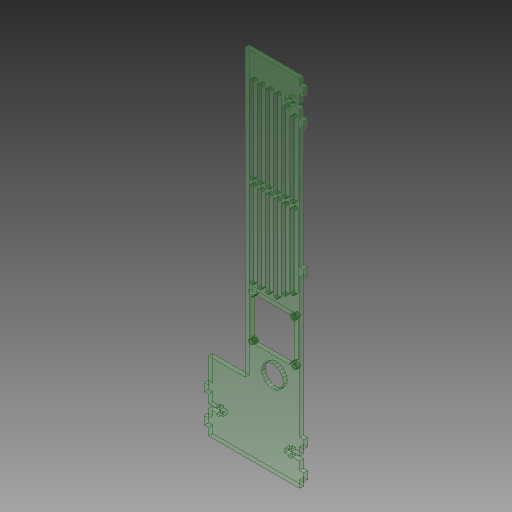
# Autodesk Inventor part: EE Side 2
Saved by Autodesk Inventor 2018 (Build 220112000, 112)
## iProperties
Created: 2016-07-27
Part Number: EE Side 2
Material: Polycarbonate, Green
Document SubType Name: Modeling
Designer: User
Density: 1.2 g/cm^3
Appearance: Polycarbonate - Clear(2)
Author: User
Autodesk Inventor part; units mm, degrees
ref_plane "YZ Plane" through (0, 0, 0) normal (1, 0, 0) x (0, 1, 0)
ref_plane "XZ Plane" through (0, 0, 0) normal (0, 1, 0) x (-1, 0, 0)
ref_plane "XY Plane" through (0, 0, 0) normal (0, 0, 1) x (1, 0, 0)
sketch "Sketch1" plane through (0, 0, 0) normal (0, 0, 1) x (1, 0, 0)
  line L0 (150.9594, -29.9434) -> (150.9594, -23.8434)
  line L1 (150.9594, -23.8434) -> (153.9594, -23.8434)
  line L2 (153.9594, -23.8434) -> (153.9594, -17.8434)
  line L3 (153.9594, -17.8434) -> (150.9594, -17.8434)
  line L4 (150.9594, -17.8434) -> (150.9594, -13.3231)
  line L5 (150.9594, -13.3231) -> (146.9594, -13.3231)
  line L6 (146.9594, -13.3231) -> (143.9594, -13.3231)
  line L7 (143.9594, -13.3231) -> (140.9594, -13.3231)
  line L8 (140.9594, -13.3231) -> (137.9594, -13.3231)
  line L9 (137.9594, -13.3231) -> (134.9594, -13.3231)
  line L10 (134.9594, -13.3231) -> (131.9593, -13.3231)
  line L11 (131.9593, -13.3231) -> (128.9594, -13.3231)
  line L12 (128.9594, -13.3231) -> (125.9593, -13.3231)
  line L13 (125.9593, -13.3231) -> (122.9594, -13.3231)
  line L14 (122.9594, -13.3231) -> (119.9594, -13.3231)
  line L15 (119.9594, -13.3231) -> (116.9593, -13.3231)
  line L16 (116.9593, -13.3231) -> (113.9593, -13.3231)
  line L17 (113.9593, -13.3231) -> (110.9594, -13.3231)
  line L18 (110.9594, -13.3231) -> (110.9594, -118.3231)
  line L19 (110.9594, -118.3231) -> (110.9594, -223.7405)
  line L20 (110.9594, -223.7405) -> (83.9593, -223.7405)
  line L21 (83.9593, -223.7405) -> (83.9593, -242.1298)
  line L22 (83.9593, -242.1298) -> (80.9594, -242.1298)
  line L23 (80.9594, -242.1298) -> (80.9594, -248.1298)
  line L24 (80.9594, -248.1298) -> (83.9593, -248.1298)
  line L25 (83.9593, -248.1298) -> (83.9593, -250.7405)
  line L26 (83.9593, -250.7405) -> (83.9593, -254.2298)
  line L27 (83.9593, -254.2298) -> (89.9593, -254.2298)
  line L28 (89.9593, -254.2298) -> (89.9593, -252.9798)
  line L29 (89.9593, -252.9798) -> (91.9594, -252.9798)
  line L30 (91.9594, -252.9798) -> (91.9594, -254.2298)
  line L31 (91.9594, -254.2298) -> (94.6093, -254.2298)
  line L32 (94.6093, -254.2298) -> (94.6093, -257.2298)
  line L33 (94.6093, -257.2298) -> (91.9594, -257.2298)
  line L34 (91.9594, -257.2298) -> (91.9594, -258.4798)
  line L35 (91.9594, -258.4798) -> (89.9593, -258.4798)
  line L36 (89.9593, -258.4798) -> (89.9593, -257.2298)
  line L37 (89.9593, -257.2298) -> (83.9593, -257.2298)
  line L38 (83.9593, -257.2298) -> (83.9593, -263.3298)
  line L39 (83.9593, -263.3298) -> (80.9594, -263.3298)
  line L40 (80.9594, -263.3298) -> (80.9594, -269.3297)
  line L41 (80.9594, -269.3297) -> (83.9593, -269.3297)
  line L42 (83.9593, -269.3297) -> (83.9593, -269.4298)
  line L43 (83.9593, -269.4298) -> (83.9593, -274.7405)
  line L44 (83.9593, -274.7405) -> (150.9594, -274.7405)
  line L45 (150.9594, -274.7405) -> (150.9594, -269.3434)
  line L46 (150.9594, -269.3434) -> (153.9594, -269.3434)
  line L47 (153.9594, -269.3434) -> (153.9594, -263.3434)
  line L48 (153.9594, -263.3434) -> (150.9594, -263.3434)
  line L49 (150.9594, -263.3434) -> (150.9594, -260.7327)
  line L50 (150.9594, -260.7327) -> (150.9594, -257.2434)
  line L51 (150.9594, -257.2434) -> (144.9593, -257.2434)
  line L52 (144.9593, -257.2434) -> (144.9593, -258.4934)
  line L53 (144.9593, -258.4934) -> (142.9593, -258.4934)
  line L54 (142.9593, -258.4934) -> (142.9593, -257.2434)
  line L55 (142.9593, -257.2434) -> (140.3094, -257.2434)
  line L56 (140.3094, -257.2434) -> (140.3094, -254.2434)
  line L57 (140.3094, -254.2434) -> (142.9593, -254.2434)
  line L58 (142.9593, -254.2434) -> (142.9593, -252.9934)
  line L59 (142.9593, -252.9934) -> (144.9593, -252.9934)
  line L60 (144.9593, -252.9934) -> (144.9593, -254.2434)
  line L61 (144.9593, -254.2434) -> (150.9594, -254.2434)
  line L62 (150.9594, -254.2434) -> (150.9594, -248.1434)
  line L63 (150.9594, -248.1434) -> (153.9594, -248.1434)
  line L64 (153.9594, -248.1434) -> (153.9594, -242.1434)
  line L65 (153.9594, -242.1434) -> (150.9594, -242.1434)
  line L66 (150.9594, -242.1434) -> (150.9594, -139.5434)
  line L67 (150.9594, -139.5434) -> (153.9594, -139.5434)
  line L68 (153.9594, -139.5434) -> (153.9594, -133.5434)
  line L69 (153.9594, -133.5434) -> (150.9594, -133.5434)
  line L70 (150.9594, -133.5434) -> (150.9594, -45.0434)
  line L71 (150.9594, -45.0434) -> (153.9594, -45.0434)
  line L72 (153.9594, -45.0434) -> (153.9594, -39.0434)
  line L73 (153.9594, -39.0434) -> (150.9594, -39.0434)
  line L74 (150.9594, -39.0434) -> (150.9594, -36.4327)
  line L75 (150.9594, -36.4327) -> (150.9594, -32.9434)
  line L76 (150.9594, -32.9434) -> (144.9593, -32.9434)
  line L77 (144.9593, -32.9434) -> (144.9593, -34.1934)
  line L78 (144.9593, -34.1934) -> (142.9593, -34.1934)
  line L79 (142.9593, -34.1934) -> (142.9593, -32.9434)
  line L80 (142.9593, -32.9434) -> (140.3094, -32.9434)
  line L81 (140.3094, -32.9434) -> (140.3094, -29.9434)
  line L82 (140.3094, -29.9434) -> (142.9593, -29.9434)
  line L83 (142.9593, -29.9434) -> (142.9593, -28.6934)
  line L84 (142.9593, -28.6934) -> (144.9593, -28.6934)
  line L85 (144.9593, -28.6934) -> (144.9593, -29.9434)
  line L86 (144.9593, -29.9434) -> (150.9594, -29.9434)
  line L87 (146.5595, -170.5352) -> (146.17, -170.4202)
  line L88 (146.17, -170.4202) -> (145.7956, -170.2628)
  line L89 (145.7956, -170.2628) -> (145.4409, -170.065)
  line L90 (145.4409, -170.065) -> (145.1102, -169.8292)
  line L91 (145.1102, -169.8292) -> (144.8075, -169.5584)
  line L92 (144.8075, -169.5584) -> (144.5367, -169.2558)
  line L93 (144.5367, -169.2558) -> (144.3009, -168.925)
  line L94 (144.3009, -168.925) -> (144.1031, -168.5703)
  line L95 (144.1031, -168.5703) -> (143.9458, -168.1959)
  line L96 (143.9458, -168.1959) -> (143.8307, -167.8064)
  line L97 (143.8307, -167.8064) -> (143.7593, -167.4066)
  line L98 (143.7593, -167.4066) -> (118.1593, -167.4066)
  line L99 (118.1593, -167.4066) -> (118.0788, -167.8022)
  line L100 (118.0788, -167.8022) -> (117.9568, -168.1871)
  line L101 (117.9568, -168.1871) -> (117.7946, -168.5569)
  line L102 (117.7946, -168.5569) -> (117.5941, -168.9073)
  line L103 (117.5941, -168.9073) -> (117.3575, -169.2346)
  line L104 (117.3575, -169.2346) -> (117.0876, -169.5348)
  line L105 (117.0876, -169.5348) -> (116.7874, -169.8048)
  line L106 (116.7874, -169.8048) -> (116.4601, -170.0413)
  line L107 (116.4601, -170.0413) -> (116.1097, -170.2418)
  line L108 (116.1097, -170.2418) -> (115.7399, -170.404)
  line L109 (115.7399, -170.404) -> (115.355, -170.5261)
  line L110 (115.355, -170.5261) -> (114.9593, -170.6066)
  line L111 (114.9593, -170.6066) -> (114.9593, -196.2066)
  line L112 (114.9593, -196.2066) -> (115.3592, -196.2779)
  line L113 (115.3592, -196.2779) -> (115.7487, -196.393)
  line L114 (115.7487, -196.393) -> (116.1231, -196.5503)
  line L115 (116.1231, -196.5503) -> (116.4778, -196.7482)
  line L116 (116.4778, -196.7482) -> (116.8085, -196.9839)
  line L117 (116.8085, -196.9839) -> (117.1111, -197.2548)
  line L118 (117.1111, -197.2548) -> (117.382, -197.5574)
  line L119 (117.382, -197.5574) -> (117.6178, -197.8881)
  line L120 (117.6178, -197.8881) -> (117.8156, -198.2428)
  line L121 (117.8156, -198.2428) -> (117.9729, -198.6172)
  line L122 (117.9729, -198.6172) -> (118.088, -199.0067)
  line L123 (118.088, -199.0067) -> (118.1593, -199.4066)
  line L124 (118.1593, -199.4066) -> (143.7593, -199.4066)
  line L125 (143.7593, -199.4066) -> (143.8399, -199.0109)
  line L126 (143.8399, -199.0109) -> (143.9619, -198.626)
  line L127 (143.9619, -198.626) -> (144.1241, -198.2563)
  line L128 (144.1241, -198.2563) -> (144.3246, -197.9058)
  line L129 (144.3246, -197.9058) -> (144.5611, -197.5786)
  line L130 (144.5611, -197.5786) -> (144.8311, -197.2783)
  line L131 (144.8311, -197.2783) -> (145.1314, -197.0084)
  line L132 (145.1314, -197.0084) -> (145.4586, -196.7718)
  line L133 (145.4586, -196.7718) -> (145.8091, -196.5713)
  line L134 (145.8091, -196.5713) -> (146.1788, -196.4091)
  line L135 (146.1788, -196.4091) -> (146.5637, -196.2871)
  line L136 (146.5637, -196.2871) -> (146.9594, -196.2066)
  line L137 (146.9594, -196.2066) -> (146.9594, -170.6066)
  line L138 (146.9594, -170.6066) -> (146.5595, -170.5352)
  line L139 (148.6014, -198.9666) -> (148.4316, -198.5566)
  line L140 (148.4316, -198.5566) -> (148.1615, -198.2045)
  line L141 (148.1615, -198.2045) -> (147.8093, -197.9343)
  line L142 (147.8093, -197.9343) -> (147.3993, -197.7645)
  line L143 (147.3993, -197.7645) -> (146.9594, -197.7066)
  line L144 (146.9594, -197.7066) -> (146.5194, -197.7645)
  line L145 (146.5194, -197.7645) -> (146.1094, -197.9343)
  line L146 (146.1094, -197.9343) -> (145.7573, -198.2045)
  line L147 (145.7573, -198.2045) -> (145.4871, -198.5566)
  line L148 (145.4871, -198.5566) -> (145.3173, -198.9666)
  line L149 (145.3173, -198.9666) -> (145.2594, -199.4066)
  line L150 (145.2594, -199.4066) -> (145.3173, -199.8466)
  line L151 (145.3173, -199.8466) -> (145.4871, -200.2566)
  line L152 (145.4871, -200.2566) -> (145.7573, -200.6087)
  line L153 (145.7573, -200.6087) -> (146.1094, -200.8788)
  line L154 (146.1094, -200.8788) -> (146.5194, -201.0486)
  line L155 (146.5194, -201.0486) -> (146.9594, -201.1066)
  line L156 (146.9594, -201.1066) -> (147.3993, -201.0486)
  line L157 (147.3993, -201.0486) -> (147.8093, -200.8788)
  line L158 (147.8093, -200.8788) -> (148.1615, -200.6087)
  line L159 (148.1615, -200.6087) -> (148.4316, -200.2566)
  line L160 (148.4316, -200.2566) -> (148.6014, -199.8466)
  line L161 (148.6014, -199.8466) -> (148.6594, -199.4066)
  line L162 (148.6594, -199.4066) -> (148.6014, -198.9666)
  line L163 (148.6014, -166.9666) -> (148.4316, -166.5566)
  line L164 (148.4316, -166.5566) -> (148.1615, -166.2045)
  line L165 (148.1615, -166.2045) -> (147.8093, -165.9344)
  line L166 (147.8093, -165.9344) -> (147.3993, -165.7645)
  line L167 (147.3993, -165.7645) -> (146.9594, -165.7066)
  line L168 (146.9594, -165.7066) -> (146.5194, -165.7645)
  line L169 (146.5194, -165.7645) -> (146.1094, -165.9344)
  line L170 (146.1094, -165.9344) -> (145.7573, -166.2045)
  line L171 (145.7573, -166.2045) -> (145.4871, -166.5566)
  line L172 (145.4871, -166.5566) -> (145.3173, -166.9666)
  line L173 (145.3173, -166.9666) -> (145.2594, -167.4066)
  line L174 (145.2594, -167.4066) -> (145.3173, -167.8466)
  line L175 (145.3173, -167.8466) -> (145.4871, -168.2566)
  line L176 (145.4871, -168.2566) -> (145.7573, -168.6087)
  line L177 (145.7573, -168.6087) -> (146.1094, -168.8788)
  line L178 (146.1094, -168.8788) -> (146.5194, -169.0486)
  line L179 (146.5194, -169.0486) -> (146.9594, -169.1066)
  line L180 (146.9594, -169.1066) -> (147.3993, -169.0486)
  line L181 (147.3993, -169.0486) -> (147.8093, -168.8788)
  line L182 (147.8093, -168.8788) -> (148.1615, -168.6087)
  line L183 (148.1615, -168.6087) -> (148.4316, -168.2566)
  line L184 (148.4316, -168.2566) -> (148.6014, -167.8466)
  line L185 (148.6014, -167.8466) -> (148.6594, -167.4066)
  line L186 (148.6594, -167.4066) -> (148.6014, -166.9666)
  line L187 (116.6014, -198.9666) -> (116.4316, -198.5566)
  line L188 (116.4316, -198.5566) -> (116.1614, -198.2045)
  line L189 (116.1614, -198.2045) -> (115.8094, -197.9343)
  line L190 (115.8094, -197.9343) -> (115.3994, -197.7645)
  line L191 (115.3994, -197.7645) -> (114.9593, -197.7066)
  line L192 (114.9593, -197.7066) -> (114.5193, -197.7645)
  line L193 (114.5193, -197.7645) -> (114.1094, -197.9343)
  line L194 (114.1094, -197.9343) -> (113.7573, -198.2045)
  line L195 (113.7573, -198.2045) -> (113.4871, -198.5566)
  line L196 (113.4871, -198.5566) -> (113.3173, -198.9666)
  line L197 (113.3173, -198.9666) -> (113.2593, -199.4066)
  line L198 (113.2593, -199.4066) -> (113.3173, -199.8466)
  line L199 (113.3173, -199.8466) -> (113.4871, -200.2566)
  line L200 (113.4871, -200.2566) -> (113.7573, -200.6087)
  line L201 (113.7573, -200.6087) -> (114.1094, -200.8788)
  line L202 (114.1094, -200.8788) -> (114.5193, -201.0486)
  line L203 (114.5193, -201.0486) -> (114.9593, -201.1066)
  line L204 (114.9593, -201.1066) -> (115.3994, -201.0486)
  line L205 (115.3994, -201.0486) -> (115.8094, -200.8788)
  line L206 (115.8094, -200.8788) -> (116.1614, -200.6087)
  line L207 (116.1614, -200.6087) -> (116.4316, -200.2566)
  line L208 (116.4316, -200.2566) -> (116.6014, -199.8466)
  line L209 (116.6014, -199.8466) -> (116.6593, -199.4066)
  line L210 (116.6593, -199.4066) -> (116.6014, -198.9666)
  line L211 (116.9082, -32.9348) -> (116.7584, -32.5731)
  line L212 (116.7584, -32.5731) -> (116.52, -32.2624)
  line L213 (116.52, -32.2624) -> (116.2093, -32.024)
  line L214 (116.2093, -32.024) -> (115.8476, -31.8742)
  line L215 (115.8476, -31.8742) -> (115.4594, -31.8231)
  line L216 (115.4594, -31.8231) -> (115.0711, -31.8742)
  line L217 (115.0711, -31.8742) -> (114.7094, -32.024)
  line L218 (114.7094, -32.024) -> (114.3987, -32.2624)
  line L219 (114.3987, -32.2624) -> (114.1603, -32.5731)
  line L220 (114.1603, -32.5731) -> (114.0105, -32.9348)
  line L221 (114.0105, -32.9348) -> (113.9593, -33.3231)
  spline S0 degree 3 poles (113.9593, -33.3231) (113.9593, -53.8006) (113.8767, -74.2899) (114.0105, -94.7613) knots 11 11 11 11 12 12 12 12
  line L222 (113.9593, -33.3231) -> (113.9593, -53.8006) construction
  line L223 (113.9593, -53.8006) -> (113.8767, -74.2899) construction
  line L224 (113.8767, -74.2899) -> (114.0105, -94.7613) construction
  line L225 (114.0105, -94.7613) -> (114.1603, -95.1231)
  line L226 (114.1603, -95.1231) -> (114.3987, -95.4337)
  line L227 (114.3987, -95.4337) -> (114.7094, -95.6721)
  line L228 (114.7094, -95.6721) -> (115.0711, -95.822)
  line L229 (115.0711, -95.822) -> (115.4594, -95.8731)
  line L230 (115.4594, -95.8731) -> (115.8476, -95.822)
  line L231 (115.8476, -95.822) -> (116.2093, -95.6721)
  line L232 (116.2093, -95.6721) -> (116.52, -95.4337)
  line L233 (116.52, -95.4337) -> (116.7584, -95.1231)
  line L234 (116.7584, -95.1231) -> (116.9082, -94.7613)
  spline S1 degree 3 poles (116.9082, -94.7613) (117.0428, -74.1633) (117.0428, -53.5328) (116.9082, -32.9348) knots 22 22 22 22 23 23 23 23
  line L235 (116.9082, -94.7613) -> (117.0428, -74.1633) construction
  line L236 (117.0428, -74.1633) -> (117.0428, -53.5328) construction
  line L237 (117.0428, -53.5328) -> (116.9082, -32.9348) construction
  line L238 (116.6014, -166.9666) -> (116.4316, -166.5566)
  line L239 (116.4316, -166.5566) -> (116.1614, -166.2045)
  line L240 (116.1614, -166.2045) -> (115.8094, -165.9344)
  line L241 (115.8094, -165.9344) -> (115.3994, -165.7645)
  line L242 (115.3994, -165.7645) -> (114.9593, -165.7066)
  line L243 (114.9593, -165.7066) -> (114.5193, -165.7645)
  line L244 (114.5193, -165.7645) -> (114.1094, -165.9344)
  line L245 (114.1094, -165.9344) -> (113.7573, -166.2045)
  line L246 (113.7573, -166.2045) -> (113.4871, -166.5566)
  line L247 (113.4871, -166.5566) -> (113.3173, -166.9666)
  line L248 (113.3173, -166.9666) -> (113.2593, -167.4066)
  line L249 (113.2593, -167.4066) -> (113.3173, -167.8466)
  line L250 (113.3173, -167.8466) -> (113.4871, -168.2566)
  line L251 (113.4871, -168.2566) -> (113.7573, -168.6087)
  line L252 (113.7573, -168.6087) -> (114.1094, -168.8788)
  line L253 (114.1094, -168.8788) -> (114.5193, -169.0486)
  line L254 (114.5193, -169.0486) -> (114.9593, -169.1066)
  line L255 (114.9593, -169.1066) -> (115.3994, -169.0486)
  line L256 (115.3994, -169.0486) -> (115.8094, -168.8788)
  line L257 (115.8094, -168.8788) -> (116.1614, -168.6087)
  line L258 (116.1614, -168.6087) -> (116.4316, -168.2566)
  line L259 (116.4316, -168.2566) -> (116.6014, -167.8466)
  line L260 (116.6014, -167.8466) -> (116.6593, -167.4066)
  line L261 (116.6593, -167.4066) -> (116.6014, -166.9666)
  line L262 (138.481, -210.5158) -> (137.5196, -208.6618)
  line L263 (137.5196, -208.6618) -> (136.111, -207.12)
  line L264 (136.111, -207.12) -> (134.3513, -205.9952)
  line L265 (134.3513, -205.9952) -> (132.3605, -205.3641)
  line L266 (132.3605, -205.3641) -> (130.2742, -205.2699)
  line L267 (130.2742, -205.2699) -> (128.2346, -205.7188)
  line L268 (128.2346, -205.7188) -> (126.3807, -206.6803)
  line L269 (126.3807, -206.6803) -> (124.8388, -208.0888)
  line L270 (124.8388, -208.0888) -> (123.714, -209.8485)
  line L271 (123.714, -209.8485) -> (123.083, -211.8393)
  line L272 (123.083, -211.8393) -> (123.0197, -213.2405)
  line L273 (123.0197, -213.2405) -> (122.9887, -213.9256)
  line L274 (122.9887, -213.9256) -> (123.4376, -215.9652)
  line L275 (123.4376, -215.9652) -> (124.3992, -217.8191)
  line L276 (124.3992, -217.8191) -> (125.8078, -219.361)
  line L277 (125.8078, -219.361) -> (127.5674, -220.4858)
  line L278 (127.5674, -220.4858) -> (129.5582, -221.1168)
  line L279 (129.5582, -221.1168) -> (131.6445, -221.2111)
  line L280 (131.6445, -221.2111) -> (133.6841, -220.7621)
  line L281 (133.6841, -220.7621) -> (135.538, -219.8007)
  line L282 (135.538, -219.8007) -> (137.0799, -218.3921)
  line L283 (137.0799, -218.3921) -> (138.2047, -216.6324)
  line L284 (138.2047, -216.6324) -> (138.8357, -214.6416)
  line L285 (138.8357, -214.6416) -> (138.93, -212.5554)
  line L286 (138.93, -212.5554) -> (138.481, -210.5158)
  line L287 (116.9082, -99.9848) -> (116.7584, -99.6231)
  line L288 (116.7584, -99.6231) -> (116.52, -99.3124)
  line L289 (116.52, -99.3124) -> (116.2093, -99.074)
  line L290 (116.2093, -99.074) -> (115.8476, -98.9242)
  line L291 (115.8476, -98.9242) -> (115.4594, -98.8731)
  line L292 (115.4594, -98.8731) -> (115.0711, -98.9242)
  line L293 (115.0711, -98.9242) -> (114.7094, -99.074)
  line L294 (114.7094, -99.074) -> (114.3987, -99.3124)
  line L295 (114.3987, -99.3124) -> (114.1603, -99.6231)
  line L296 (114.1603, -99.6231) -> (114.0105, -99.9848)
  spline S2 degree 3 poles (114.0105, -99.9848) (113.8759, -120.5674) (113.8759, -141.1826) (114.0105, -161.7651) knots 10 10 10 10 11 11 11 11
  line L297 (114.0105, -99.9848) -> (113.8759, -120.5674) construction
  line L298 (113.8759, -120.5674) -> (113.8759, -141.1826) construction
  line L299 (113.8759, -141.1826) -> (114.0105, -161.7651) construction
  line L300 (114.0105, -161.7651) -> (114.1603, -162.1269)
  line L301 (114.1603, -162.1269) -> (114.3987, -162.4375)
  line L302 (114.3987, -162.4375) -> (114.7094, -162.6759)
  line L303 (114.7094, -162.6759) -> (115.0711, -162.8258)
  line L304 (115.0711, -162.8258) -> (115.4594, -162.8769)
  line L305 (115.4594, -162.8769) -> (115.8476, -162.8258)
  line L306 (115.8476, -162.8258) -> (116.2093, -162.6759)
  line L307 (116.2093, -162.6759) -> (116.52, -162.4375)
  line L308 (116.52, -162.4375) -> (116.7584, -162.1269)
  line L309 (116.7584, -162.1269) -> (116.9082, -161.7651)
  line L310 (116.9082, -161.7651) -> (116.9593, -161.3769)
  spline S3 degree 3 poles (116.9593, -161.3769) (116.9593, -140.9148) (117.042, -120.4409) (116.9082, -99.9848) knots 22 22 22 22 23 23 23 23
  line L311 (116.9593, -161.3769) -> (116.9593, -140.9148) construction
  line L312 (116.9593, -140.9148) -> (117.042, -120.4409) construction
  line L313 (117.042, -120.4409) -> (116.9082, -99.9848) construction
  line L314 (122.9082, -99.9848) -> (122.7584, -99.6231)
  line L315 (122.7584, -99.6231) -> (122.52, -99.3124)
  line L316 (122.52, -99.3124) -> (122.2094, -99.074)
  line L317 (122.2094, -99.074) -> (121.8476, -98.9242)
  line L318 (121.8476, -98.9242) -> (121.4593, -98.8731)
  line L319 (121.4593, -98.8731) -> (121.0711, -98.9242)
  line L320 (121.0711, -98.9242) -> (120.7094, -99.074)
  line L321 (120.7094, -99.074) -> (120.3987, -99.3124)
  line L322 (120.3987, -99.3124) -> (120.1603, -99.6231)
  line L323 (120.1603, -99.6231) -> (120.0105, -99.9848)
  spline S4 degree 3 poles (120.0105, -99.9848) (119.8759, -120.5674) (119.8759, -141.1826) (120.0105, -161.7651) knots 10 10 10 10 11 11 11 11
  line L324 (120.0105, -99.9848) -> (119.8759, -120.5674) construction
  line L325 (119.8759, -120.5674) -> (119.8759, -141.1826) construction
  line L326 (119.8759, -141.1826) -> (120.0105, -161.7651) construction
  line L327 (120.0105, -161.7651) -> (120.1603, -162.1269)
  line L328 (120.1603, -162.1269) -> (120.3987, -162.4375)
  line L329 (120.3987, -162.4375) -> (120.7094, -162.6759)
  line L330 (120.7094, -162.6759) -> (121.0711, -162.8258)
  line L331 (121.0711, -162.8258) -> (121.4593, -162.8769)
  line L332 (121.4593, -162.8769) -> (121.8476, -162.8258)
  line L333 (121.8476, -162.8258) -> (122.2094, -162.6759)
  line L334 (122.2094, -162.6759) -> (122.52, -162.4375)
  line L335 (122.52, -162.4375) -> (122.7584, -162.1269)
  line L336 (122.7584, -162.1269) -> (122.9082, -161.7651)
  line L337 (122.9082, -161.7651) -> (122.9594, -161.3769)
  spline S5 degree 3 poles (122.9594, -161.3769) (122.9594, -140.9148) (123.042, -120.4409) (122.9082, -99.9848) knots 22 22 22 22 23 23 23 23
  line L338 (122.9594, -161.3769) -> (122.9594, -140.9148) construction
  line L339 (122.9594, -140.9148) -> (123.042, -120.4409) construction
  line L340 (123.042, -120.4409) -> (122.9082, -99.9848) construction
  line L341 (128.9082, -99.9848) -> (128.7584, -99.6231)
  line L342 (128.7584, -99.6231) -> (128.52, -99.3124)
  line L343 (128.52, -99.3124) -> (128.2094, -99.074)
  line L344 (128.2094, -99.074) -> (127.8476, -98.9242)
  line L345 (127.8476, -98.9242) -> (127.4594, -98.8731)
  line L346 (127.4594, -98.8731) -> (127.0711, -98.9242)
  line L347 (127.0711, -98.9242) -> (126.7093, -99.074)
  line L348 (126.7093, -99.074) -> (126.3987, -99.3124)
  line L349 (126.3987, -99.3124) -> (126.1603, -99.6231)
  line L350 (126.1603, -99.6231) -> (126.0105, -99.9848)
  spline S6 degree 3 poles (126.0105, -99.9848) (125.8759, -120.5674) (125.8759, -141.1826) (126.0105, -161.7651) knots 10 10 10 10 11 11 11 11
  line L351 (126.0105, -99.9848) -> (125.8759, -120.5674) construction
  line L352 (125.8759, -120.5674) -> (125.8759, -141.1826) construction
  line L353 (125.8759, -141.1826) -> (126.0105, -161.7651) construction
  line L354 (126.0105, -161.7651) -> (126.1603, -162.1269)
  line L355 (126.1603, -162.1269) -> (126.3987, -162.4375)
  line L356 (126.3987, -162.4375) -> (126.7093, -162.6759)
  line L357 (126.7093, -162.6759) -> (127.0711, -162.8258)
  line L358 (127.0711, -162.8258) -> (127.4594, -162.8769)
  line L359 (127.4594, -162.8769) -> (127.8476, -162.8258)
  line L360 (127.8476, -162.8258) -> (128.2094, -162.6759)
  line L361 (128.2094, -162.6759) -> (128.52, -162.4375)
  line L362 (128.52, -162.4375) -> (128.7584, -162.1269)
  line L363 (128.7584, -162.1269) -> (128.9082, -161.7651)
  line L364 (128.9082, -161.7651) -> (128.9594, -161.3769)
  spline S7 degree 3 poles (128.9594, -161.3769) (128.9594, -140.9148) (129.042, -120.4409) (128.9082, -99.9848) knots 22 22 22 22 23 23 23 23
  line L365 (128.9594, -161.3769) -> (128.9594, -140.9148) construction
  line L366 (128.9594, -140.9148) -> (129.042, -120.4409) construction
  line L367 (129.042, -120.4409) -> (128.9082, -99.9848) construction
  line L368 (122.9082, -32.9348) -> (122.7584, -32.5731)
  line L369 (122.7584, -32.5731) -> (122.52, -32.2624)
  line L370 (122.52, -32.2624) -> (122.2094, -32.024)
  line L371 (122.2094, -32.024) -> (121.8476, -31.8742)
  line L372 (121.8476, -31.8742) -> (121.4593, -31.8231)
  line L373 (121.4593, -31.8231) -> (121.0711, -31.8742)
  line L374 (121.0711, -31.8742) -> (120.7094, -32.024)
  line L375 (120.7094, -32.024) -> (120.3987, -32.2624)
  line L376 (120.3987, -32.2624) -> (120.1603, -32.5731)
  line L377 (120.1603, -32.5731) -> (120.0105, -32.9348)
  spline S8 degree 3 poles (120.0105, -32.9348) (119.8759, -53.5328) (119.8759, -74.1633) (120.0105, -94.7613) knots 10 10 10 10 11 11 11 11
  line L378 (120.0105, -32.9348) -> (119.8759, -53.5328) construction
  line L379 (119.8759, -53.5328) -> (119.8759, -74.1633) construction
  line L380 (119.8759, -74.1633) -> (120.0105, -94.7613) construction
  line L381 (120.0105, -94.7613) -> (120.1603, -95.1231)
  line L382 (120.1603, -95.1231) -> (120.3987, -95.4337)
  line L383 (120.3987, -95.4337) -> (120.7094, -95.6721)
  line L384 (120.7094, -95.6721) -> (121.0711, -95.822)
  line L385 (121.0711, -95.822) -> (121.4593, -95.8731)
  line L386 (121.4593, -95.8731) -> (121.8476, -95.822)
  line L387 (121.8476, -95.822) -> (122.2094, -95.6721)
  line L388 (122.2094, -95.6721) -> (122.52, -95.4337)
  line L389 (122.52, -95.4337) -> (122.7584, -95.1231)
  line L390 (122.7584, -95.1231) -> (122.9082, -94.7613)
  spline S9 degree 3 poles (122.9082, -94.7613) (123.0428, -74.1633) (123.0428, -53.5328) (122.9082, -32.9348) knots 21 21 21 21 22 22 22 22
  line L391 (122.9082, -94.7613) -> (123.0428, -74.1633) construction
  line L392 (123.0428, -74.1633) -> (123.0428, -53.5328) construction
  line L393 (123.0428, -53.5328) -> (122.9082, -32.9348) construction
  line L394 (134.9083, -99.9848) -> (134.7584, -99.6231)
  line L395 (134.7584, -99.6231) -> (134.52, -99.3124)
  line L396 (134.52, -99.3124) -> (134.2094, -99.074)
  line L397 (134.2094, -99.074) -> (133.8476, -98.9242)
  line L398 (133.8476, -98.9242) -> (133.4594, -98.8731)
  line L399 (133.4594, -98.8731) -> (133.0711, -98.9242)
  line L400 (133.0711, -98.9242) -> (132.7094, -99.074)
  line L401 (132.7094, -99.074) -> (132.3987, -99.3124)
  line L402 (132.3987, -99.3124) -> (132.1603, -99.6231)
  line L403 (132.1603, -99.6231) -> (132.0105, -99.9848)
  spline S10 degree 3 poles (132.0105, -99.9848) (131.8759, -120.5674) (131.8759, -141.1826) (132.0105, -161.7651) knots 10 10 10 10 11 11 11 11
  line L404 (132.0105, -99.9848) -> (131.8759, -120.5674) construction
  line L405 (131.8759, -120.5674) -> (131.8759, -141.1826) construction
  line L406 (131.8759, -141.1826) -> (132.0105, -161.7651) construction
  line L407 (132.0105, -161.7651) -> (132.1603, -162.1269)
  line L408 (132.1603, -162.1269) -> (132.3987, -162.4375)
  line L409 (132.3987, -162.4375) -> (132.7094, -162.6759)
  line L410 (132.7094, -162.6759) -> (133.0711, -162.8258)
  line L411 (133.0711, -162.8258) -> (133.4594, -162.8769)
  line L412 (133.4594, -162.8769) -> (133.8476, -162.8258)
  line L413 (133.8476, -162.8258) -> (134.2094, -162.6759)
  line L414 (134.2094, -162.6759) -> (134.52, -162.4375)
  line L415 (134.52, -162.4375) -> (134.7584, -162.1269)
  line L416 (134.7584, -162.1269) -> (134.9083, -161.7651)
  line L417 (134.9083, -161.7651) -> (134.9594, -161.3769)
  spline S11 degree 3 poles (134.9594, -161.3769) (134.9594, -140.9148) (135.042, -120.4409) (134.9083, -99.9848) knots 22 22 22 22 23 23 23 23
  line L418 (134.9594, -161.3769) -> (134.9594, -140.9148) construction
  line L419 (134.9594, -140.9148) -> (135.042, -120.4409) construction
  line L420 (135.042, -120.4409) -> (134.9083, -99.9848) construction
  line L421 (128.9082, -32.9348) -> (128.7584, -32.5731)
  line L422 (128.7584, -32.5731) -> (128.52, -32.2624)
  line L423 (128.52, -32.2624) -> (128.2094, -32.024)
  line L424 (128.2094, -32.024) -> (127.8476, -31.8742)
  line L425 (127.8476, -31.8742) -> (127.4594, -31.8231)
  line L426 (127.4594, -31.8231) -> (127.0711, -31.8742)
  line L427 (127.0711, -31.8742) -> (126.7093, -32.024)
  line L428 (126.7093, -32.024) -> (126.3987, -32.2624)
  line L429 (126.3987, -32.2624) -> (126.1603, -32.5731)
  line L430 (126.1603, -32.5731) -> (126.0105, -32.9348)
  spline S12 degree 3 poles (126.0105, -32.9348) (125.8759, -53.5328) (125.8759, -74.1633) (126.0105, -94.7613) knots 10 10 10 10 11 11 11 11
  line L431 (126.0105, -32.9348) -> (125.8759, -53.5328) construction
  line L432 (125.8759, -53.5328) -> (125.8759, -74.1633) construction
  line L433 (125.8759, -74.1633) -> (126.0105, -94.7613) construction
  line L434 (126.0105, -94.7613) -> (126.1603, -95.1231)
  line L435 (126.1603, -95.1231) -> (126.3987, -95.4337)
  line L436 (126.3987, -95.4337) -> (126.7093, -95.6721)
  line L437 (126.7093, -95.6721) -> (127.0711, -95.822)
  line L438 (127.0711, -95.822) -> (127.4594, -95.8731)
  line L439 (127.4594, -95.8731) -> (127.8476, -95.822)
  line L440 (127.8476, -95.822) -> (128.2094, -95.6721)
  line L441 (128.2094, -95.6721) -> (128.52, -95.4337)
  line L442 (128.52, -95.4337) -> (128.7584, -95.1231)
  line L443 (128.7584, -95.1231) -> (128.9082, -94.7613)
  spline S13 degree 3 poles (128.9082, -94.7613) (129.0428, -74.1633) (129.0428, -53.5328) (128.9082, -32.9348) knots 21 21 21 21 22 22 22 22
  line L444 (128.9082, -94.7613) -> (129.0428, -74.1633) construction
  line L445 (129.0428, -74.1633) -> (129.0428, -53.5328) construction
  line L446 (129.0428, -53.5328) -> (128.9082, -32.9348) construction
  line L447 (146.9082, -41.1504) -> (146.7584, -40.8031)
  line L448 (146.7584, -40.8031) -> (146.52, -40.5048)
  line L449 (146.52, -40.5048) -> (146.2094, -40.276)
  line L450 (146.2094, -40.276) -> (145.8476, -40.1321)
  line L451 (145.8476, -40.1321) -> (145.4593, -40.0831)
  line L452 (145.4593, -40.0831) -> (145.0711, -40.1321)
  line L453 (145.0711, -40.1321) -> (144.7093, -40.276)
  line L454 (144.7093, -40.276) -> (144.3987, -40.5048)
  line L455 (144.3987, -40.5048) -> (144.1603, -40.8031)
  line L456 (144.1603, -40.8031) -> (144.0105, -41.1504)
  line L457 (144.0105, -41.1504) -> (143.9594, -41.5231)
  spline S14 degree 3 poles (143.9594, -41.5231) (143.9594, -59.2674) (143.8965, -77.023) (144.0105, -94.7613) knots 11 11 11 11 12 12 12 12
  line L458 (143.9594, -41.5231) -> (143.9594, -59.2674) construction
  line L459 (143.9594, -59.2674) -> (143.8965, -77.023) construction
  line L460 (143.8965, -77.023) -> (144.0105, -94.7613) construction
  line L461 (144.0105, -94.7613) -> (144.1603, -95.1231)
  line L462 (144.1603, -95.1231) -> (144.3987, -95.4337)
  line L463 (144.3987, -95.4337) -> (144.7093, -95.6721)
  line L464 (144.7093, -95.6721) -> (145.0711, -95.822)
  line L465 (145.0711, -95.822) -> (145.4593, -95.8731)
  line L466 (145.4593, -95.8731) -> (145.8476, -95.822)
  line L467 (145.8476, -95.822) -> (146.2094, -95.6721)
  line L468 (146.2094, -95.6721) -> (146.52, -95.4337)
  line L469 (146.52, -95.4337) -> (146.7584, -95.1231)
  line L470 (146.7584, -95.1231) -> (146.9082, -94.7613)
  spline S15 degree 3 poles (146.9082, -94.7613) (147.0231, -76.9012) (147.023, -59.0102) (146.9082, -41.1504) knots 22 22 22 22 23 23 23 23
  line L471 (146.9082, -94.7613) -> (147.0231, -76.9012) construction
  line L472 (147.0231, -76.9012) -> (147.023, -59.0102) construction
  line L473 (147.023, -59.0102) -> (146.9082, -41.1504) construction
  line L474 (134.9083, -32.9348) -> (134.7584, -32.5731)
  line L475 (134.7584, -32.5731) -> (134.52, -32.2624)
  line L476 (134.52, -32.2624) -> (134.2094, -32.024)
  line L477 (134.2094, -32.024) -> (133.8476, -31.8742)
  line L478 (133.8476, -31.8742) -> (133.4594, -31.8231)
  line L479 (133.4594, -31.8231) -> (133.0711, -31.8742)
  line L480 (133.0711, -31.8742) -> (132.7094, -32.024)
  line L481 (132.7094, -32.024) -> (132.3987, -32.2624)
  line L482 (132.3987, -32.2624) -> (132.1603, -32.5731)
  line L483 (132.1603, -32.5731) -> (132.0105, -32.9348)
  spline S16 degree 3 poles (132.0105, -32.9348) (131.8759, -53.5328) (131.8759, -74.1633) (132.0105, -94.7613) knots 10 10 10 10 11 11 11 11
  line L484 (132.0105, -32.9348) -> (131.8759, -53.5328) construction
  line L485 (131.8759, -53.5328) -> (131.8759, -74.1633) construction
  line L486 (131.8759, -74.1633) -> (132.0105, -94.7613) construction
  line L487 (132.0105, -94.7613) -> (132.1603, -95.1231)
  line L488 (132.1603, -95.1231) -> (132.3987, -95.4337)
  line L489 (132.3987, -95.4337) -> (132.7094, -95.6721)
  line L490 (132.7094, -95.6721) -> (133.0711, -95.822)
  line L491 (133.0711, -95.822) -> (133.4594, -95.8731)
  line L492 (133.4594, -95.8731) -> (133.8476, -95.822)
  line L493 (133.8476, -95.822) -> (134.2094, -95.6721)
  line L494 (134.2094, -95.6721) -> (134.52, -95.4337)
  line L495 (134.52, -95.4337) -> (134.7584, -95.1231)
  line L496 (134.7584, -95.1231) -> (134.9083, -94.7613)
  spline S17 degree 3 poles (134.9083, -94.7613) (135.0429, -74.1633) (135.0429, -53.5328) (134.9083, -32.9348) knots 21 21 21 21 22 22 22 22
  line L497 (134.9083, -94.7613) -> (135.0429, -74.1633) construction
  line L498 (135.0429, -74.1633) -> (135.0429, -53.5328) construction
  line L499 (135.0429, -53.5328) -> (134.9083, -32.9348) construction
  line L500 (140.9082, -37.9349) -> (140.7584, -37.5731)
  line L501 (140.7584, -37.5731) -> (140.52, -37.2624)
  line L502 (140.52, -37.2624) -> (140.2093, -37.024)
  line L503 (140.2093, -37.024) -> (139.8476, -36.8742)
  line L504 (139.8476, -36.8742) -> (139.4594, -36.8231)
  line L505 (139.4594, -36.8231) -> (139.0711, -36.8742)
  line L506 (139.0711, -36.8742) -> (138.7094, -37.024)
  line L507 (138.7094, -37.024) -> (138.3987, -37.2624)
  line L508 (138.3987, -37.2624) -> (138.1603, -37.5731)
  line L509 (138.1603, -37.5731) -> (138.0105, -37.9349)
  spline S18 degree 3 poles (138.0105, -37.9349) (137.8464, -56.864) (137.8464, -75.8321) (138.0105, -94.7613) knots 10 10 10 10 11 11 11 11
  line L510 (138.0105, -37.9349) -> (137.8464, -56.864) construction
  line L511 (137.8464, -56.864) -> (137.8464, -75.8321) construction
  line L512 (137.8464, -75.8321) -> (138.0105, -94.7613) construction
  line L513 (138.0105, -94.7613) -> (138.1603, -95.1231)
  line L514 (138.1603, -95.1231) -> (138.3987, -95.4337)
  line L515 (138.3987, -95.4337) -> (138.7094, -95.6721)
  line L516 (138.7094, -95.6721) -> (139.0711, -95.822)
  line L517 (139.0711, -95.822) -> (139.4594, -95.8731)
  line L518 (139.4594, -95.8731) -> (139.8476, -95.822)
  line L519 (139.8476, -95.822) -> (140.2093, -95.6721)
  line L520 (140.2093, -95.6721) -> (140.52, -95.4337)
  line L521 (140.52, -95.4337) -> (140.7584, -95.1231)
  line L522 (140.7584, -95.1231) -> (140.9082, -94.7613)
  spline S19 degree 3 poles (140.9082, -94.7613) (141.0723, -75.8321) (141.0723, -56.864) (140.9082, -37.9349) knots 21 21 21 21 22 22 22 22
  line L523 (140.9082, -94.7613) -> (141.0723, -75.8321) construction
  line L524 (141.0723, -75.8321) -> (141.0723, -56.864) construction
  line L525 (141.0723, -56.864) -> (140.9082, -37.9349) construction
  line L526 (140.9082, -99.9848) -> (140.7584, -99.6231)
  line L527 (140.7584, -99.6231) -> (140.52, -99.3124)
  line L528 (140.52, -99.3124) -> (140.2093, -99.074)
  line L529 (140.2093, -99.074) -> (139.8476, -98.9242)
  line L530 (139.8476, -98.9242) -> (139.4594, -98.8731)
  line L531 (139.4594, -98.8731) -> (139.0711, -98.9242)
  line L532 (139.0711, -98.9242) -> (138.7094, -99.074)
  line L533 (138.7094, -99.074) -> (138.3987, -99.3124)
  line L534 (138.3987, -99.3124) -> (138.1603, -99.6231)
  line L535 (138.1603, -99.6231) -> (138.0105, -99.9848)
  spline S20 degree 3 poles (138.0105, -99.9848) (137.8464, -118.8986) (137.8464, -137.8514) (138.0105, -156.7651) knots 10 10 10 10 11 11 11 11
  line L536 (138.0105, -99.9848) -> (137.8464, -118.8986) construction
  line L537 (137.8464, -118.8986) -> (137.8464, -137.8514) construction
  line L538 (137.8464, -137.8514) -> (138.0105, -156.7651) construction
  line L539 (138.0105, -156.7651) -> (138.1603, -157.1269)
  line L540 (138.1603, -157.1269) -> (138.3987, -157.4375)
  line L541 (138.3987, -157.4375) -> (138.7094, -157.6759)
  line L542 (138.7094, -157.6759) -> (139.0711, -157.8258)
  line L543 (139.0711, -157.8258) -> (139.4594, -157.8769)
  line L544 (139.4594, -157.8769) -> (139.8476, -157.8258)
  line L545 (139.8476, -157.8258) -> (140.2093, -157.6759)
  line L546 (140.2093, -157.6759) -> (140.52, -157.4375)
  line L547 (140.52, -157.4375) -> (140.7584, -157.1269)
  line L548 (140.7584, -157.1269) -> (140.9082, -156.7651)
  line L549 (140.9082, -156.7651) -> (140.9594, -156.3769)
  spline S21 degree 3 poles (140.9594, -156.3769) (140.9594, -137.5819) (141.0712, -118.7735) (140.9082, -99.9848) knots 22 22 22 22 23 23 23 23
  line L550 (140.9594, -156.3769) -> (140.9594, -137.5819) construction
  line L551 (140.9594, -137.5819) -> (141.0712, -118.7735) construction
  line L552 (141.0712, -118.7735) -> (140.9082, -99.9848) construction
  line L553 (146.9082, -99.9848) -> (146.7584, -99.6231)
  line L554 (146.7584, -99.6231) -> (146.52, -99.3124)
  line L555 (146.52, -99.3124) -> (146.2094, -99.074)
  line L556 (146.2094, -99.074) -> (145.8476, -98.9242)
  line L557 (145.8476, -98.9242) -> (145.4593, -98.8731)
  line L558 (145.4593, -98.8731) -> (145.0711, -98.9242)
  line L559 (145.0711, -98.9242) -> (144.7093, -99.074)
  line L560 (144.7093, -99.074) -> (144.3987, -99.3124)
  line L561 (144.3987, -99.3124) -> (144.1603, -99.6231)
  line L562 (144.1603, -99.6231) -> (144.0105, -99.9848)
  spline S22 degree 3 poles (144.0105, -99.9848) (143.8957, -117.8296) (143.8957, -135.7051) (144.0105, -153.5496) knots 10 10 10 10 11 11 11 11
  line L563 (144.0105, -99.9848) -> (143.8957, -117.8296) construction
  line L564 (143.8957, -117.8296) -> (143.8957, -135.7051) construction
  line L565 (143.8957, -135.7051) -> (144.0105, -153.5496) construction
  line L566 (144.0105, -153.5496) -> (144.1603, -153.8969)
  line L567 (144.1603, -153.8969) -> (144.3987, -154.1951)
  line L568 (144.3987, -154.1951) -> (144.7093, -154.424)
  line L569 (144.7093, -154.424) -> (145.0711, -154.5678)
  line L570 (145.0711, -154.5678) -> (145.4593, -154.6169)
  line L571 (145.4593, -154.6169) -> (145.8476, -154.5678)
  line L572 (145.8476, -154.5678) -> (146.2094, -154.424)
  line L573 (146.2094, -154.424) -> (146.52, -154.1951)
  line L574 (146.52, -154.1951) -> (146.7584, -153.8969)
  line L575 (146.7584, -153.8969) -> (146.9082, -153.5496)
  spline S23 degree 3 poles (146.9082, -153.5496) (147.023, -135.7051) (147.0231, -117.8296) (146.9082, -99.9848) knots 21 21 21 21 22 22 22 22
  line L576 (146.9082, -153.5496) -> (147.023, -135.7051) construction
  line L577 (147.023, -135.7051) -> (147.0231, -117.8296) construction
  line L578 (147.0231, -117.8296) -> (146.9082, -99.9848) construction
  point P0 (0, 0)
  constraints: 1014 end point, 72 other
extrude "Extrusion1" add sketch "Sketch1" along normal blind 3
sketch "Sketch2" plane through (0, 0, 3) normal (0, 0, 1) x (1, 0, 0)
  line L0 (116.1614, -166.2045) -> (116.4316, -166.5566) projected
  line L1 (113.3173, -167.8466) -> (113.2593, -167.4066) projected
  line L2 (114.9593, -169.1066) -> (114.5193, -169.0486) projected
  circle A0 centre (114.9593, -167.4066) radius 1.6855
  point P0 (0, 0)
  constraints: 3 tangent, 1 centre point
hole "Hole1" at (114.9593, -167.4066, 3) direction (0, 0, -1) diameter 3.4 end through all
body "Solid1"
